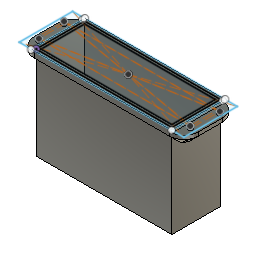
Aerostar Dash Bin Cubby v3 (Autodesk Fusion 360 design; units mm, degrees)
Autodesk Fusion 360 part; units mm, degrees
sketch "Sketch1" plane through (0, 0, 0) normal (0, 0, 1) x (1, 0, 0)
  line L0 (0, 0) -> (183, 0)
  line L1 (183, 0) -> (183, 65.4)
  line L2 (183, 65.4) -> (0, 65.4)
  line L3 (0, 65.4) -> (0, 0)
  line L4 (3.3, 62.1) -> (3.3, 3.3)
  line L5 (3.3, 3.3) -> (179.7, 3.3)
  line L6 (179.7, 3.3) -> (179.7, 62.1)
  line L7 (179.7, 62.1) -> (3.3, 62.1)
  line L8 (196.5, 51.2) -> (-13.5, 51.2) construction
  line L9 (-13.5, 51.2) -> (-13.5, 14.2) construction
  line L10 (-13.5, 14.2) -> (196.5, 14.2) construction
  line L11 (196.5, 14.2) -> (196.5, 51.2) construction
  line L12 (196.5, 51.2) -> (-13.5, 14.2) construction
  line L13 (-13.5, 51.2) -> (196.5, 14.2) construction
  line L14 (193.5, 51.2) -> (-10.5, 51.2) construction
  line L15 (-10.5, 51.2) -> (-10.5, 14.2) construction
  line L16 (-10.5, 14.2) -> (193.5, 14.2) construction
  line L17 (193.5, 14.2) -> (193.5, 51.2) construction
  line L18 (193.5, 51.2) -> (-10.5, 14.2) construction
  line L19 (-10.5, 51.2) -> (193.5, 14.2) construction
  circle A0 centre (-13.5, 51.2) radius 3.1
  circle A1 centre (196.5, 51.2) radius 3.1
  circle A2 centre (-10.5, 14.2) radius 3.1
  circle A3 centre (193.5, 14.2) radius 3.1
  line L20 (183, 65.4) -> (186, 65.4) construction
  line L21 (0, 65.4) -> (-3, 65.4) construction
  line L22 (186, 68.7) -> (186, -3.3)
  line L23 (-3, 68.7) -> (-3, -4)
  line L24 (202.5, 68.7) -> (-19.5, 68.7)
  line L25 (-19.5, 68.7) -> (-19.5, -3.3)
  line L26 (-19.5, -3.3) -> (202.5, -3.3)
  line L27 (202.5, -3.3) -> (202.5, 68.7)
  line L28 (202.5, 68.7) -> (-19.5, -3.3) construction
  line L29 (-19.5, 68.7) -> (202.5, -3.3) construction
  point P0 (91.5, 32.7)
  point P1 (91.5, 32.7)
  point P2 (91.5, 32.7)
  point P3 (91.5, 32.7)
  dimension "d1" = 65.4
  dimension "d2" = 183
  dimension "d3" = 3.3
  dimension "d4" = 37
  dimension "d5" = 204
  dimension "d6" = 6.2
  dimension "d7" = 6.2
  dimension "d8" = 6.2
  dimension "d9" = 6.2
  dimension "d20" = 3
  dimension "d21" = 3
  dimension "d26" = 222
  dimension "d27" = 72
  constraint horizontal L0
  constraint vertical L1
  constraint horizontal L2
  constraint vertical L3
  constraint coincident L0.start L3.end
  constraint perpendicular L8 L9
  constraint parallel L8 L10
  constraint parallel L9 L11
  constraint horizontal L8
  constraint coincident L12 P3
  constraint coincident L13 P3
  constraint perpendicular L14 L15
  constraint parallel L14 L16
  constraint parallel L15 L17
  constraint horizontal L14
  constraint coincident L18 P3
  constraint coincident L19 P3
  constraint coincident P3 P2
  constraint coincident L8.end L9.start
  constraint coincident L8.start L11.end
  constraint coincident L15.end L16.start
  constraint coincident L16.end L17.start
  constraint perpendicular L24 L25
  constraint parallel L24 L26
  constraint parallel L25 L27
  constraint horizontal L24
  constraint coincident L28 P3
  constraint coincident L29 P3
  measures "d1" distance of L0.start L2.end
  measures "d2" distance of L0.start L0.end
  measures "d4" distance of L8.end L9.end
  measures "d5" distance of L15.end L16.end
  measures "d6" diameter of A0
  measures "d7" diameter of A1
  measures "d8" diameter of A2
  measures "d9" diameter of A3
  measures "d20" distance of L1.end L20.end
  measures "d21" distance of L2.end L21.end
  measures "d26" distance of L25.end L26.end
  measures "d27" distance of L24.end L25.end
extrude "Extrude1" add sketch "Sketch1" against normal blind 125 contours L0 L1 L2 L3
extrude "Extrude2" add sketch "Sketch1" against normal blind 7.4 contours L22 L24 L26 L27 | L22 L23 L24 L26 | L23 L24 L25 L26
extrude "Extrude3" cut sketch "Sketch1" against normal blind 3.5 contours A0 | A2 | L22 L24 L26 L27 | L23 L24 L25 L26
sketch "Sketch2" plane through (0, 0, -125) normal (0, 0, -1) x (1, 0, 0)
  line L0 (179.7, -62.1) -> (3.3, -62.1)
  line L1 (3.3, -62.1) -> (3.3, -3.3)
  line L2 (3.3, -3.3) -> (179.7, -3.3)
  line L3 (179.7, -3.3) -> (179.7, -62.1)
  line L4 (0, 0) -> (0, -65.4)
  line L5 (0, -65.4) -> (183, -65.4)
  line L6 (183, -65.4) -> (183, 0)
  line L7 (183, 0) -> (0, 0)
  line L8 (3.3, -62.1) -> (3.3, -3.3)
  line L9 (3.3, -3.3) -> (179.7, -3.3)
  line L10 (179.7, -62.1) -> (3.3, -62.1)
  line L11 (179.7, -3.3) -> (179.7, -62.1)
extrude "Extrude4" add sketch "Sketch2" against normal blind 3.3 contours L0 L1 L2 L3 L8 L9 L10 L11
fillet "Fillet1" radius 20 4 edges at (202.5, 68.7, -5.45) (202.5, -3.3, -5.45) (-19.5, 68.7, -5.45) (-19.5, -3.3, -5.45)
extrude "Extrude5" add 1 faces at (189.1588, 43.8775, -7.4) along direction (0, 0, -1) blind 15
sketch "Sketch3" plane through (0, 0, -22.4) normal (0, 0, -1) x (1, 0, 0)
  arc A0 (0.5, 3.3) -> (-19.5, -16.7) centre (0.5, -16.7) ccw
  line L0 (-19.5, -16.7) -> (-19.5, -48.7)
  arc A1 (-19.5, -48.7) -> (0.5, -68.7) centre (0.5, -48.7) ccw
  line L1 (0.5, -68.7) -> (182.5, -68.7)
  arc A2 (182.5, -68.7) -> (202.5, -48.7) centre (182.5, -48.7) ccw
  line L2 (202.5, -48.7) -> (202.5, -16.7)
  arc A3 (202.5, -16.7) -> (182.5, 3.3) centre (182.5, -16.7) ccw
  line L3 (182.5, 3.3) -> (0.5, 3.3)
  circle A4 centre (196.5, -51.2) radius 3.1
  line L4 (0, -65.4) -> (0, 0)
  line L5 (0, 0) -> (183, 0)
  line L6 (183, 0) -> (183, -65.4)
  line L7 (183, -65.4) -> (0, -65.4)
  circle A5 centre (-13.5, -51.2) radius 3.1
  circle A6 centre (193.5, -14.2) radius 3.1
  circle A7 centre (-10.5, -14.2) radius 3.1
  circle A8 centre (196.5, -51.2) radius 6.5
  circle A9 centre (193.5, -14.2) radius 6.5
  circle A10 centre (-10.5, -14.2) radius 6.5
  circle A11 centre (-13.5, -51.2) radius 6.5
  dimension "d31" = 13
  dimension "d32" = 13
  dimension "d33" = 13
  dimension "d34" = 13
  constraint concentric A4 A8
  constraint concentric A6 A9
  constraint concentric A7 A10
  constraint concentric A5 A11
  measures "d31" diameter of A8
  measures "d32" diameter of A9
  measures "d33" diameter of A10
  measures "d34" diameter of A11
extrude "Extrude6" cut sketch "Sketch3" against normal blind 13 contours A1 A11 | A2 A8 | A9 | A10 picked at (-18.4412, -50.0123) picked at (201.4412, -50.0123)
chamfer "Chamfer1" distance 14 distance2 14 8 edges at (202.5, 32.7, -22.4) (196.6421, 2.5579, -22.4) (91.5, -3.3, -22.4) (-13.6421, 2.5579, -22.4) (-19.5, 32.7, -22.4) (-10.9359, 65.108, -22.4) (91.5, 68.7, -22.4) (193.9359, 65.108, -22.4) measured on face at (186.9487, 44.0037, -22.4) measured on face at (186.9487, 44.0037, -22.4) measured on face at (186.9487, 44.0037, -22.4) measured on face at (186.9487, 44.0037, -22.4) measured on face at (186.9487, 44.0037, -22.4) measured on face at (186.9487, 44.0037, -22.4) measured on face at (186.9487, 44.0037, -22.4) measured on face at (186.9487, 44.0037, -22.4)
equation "d3 = 7 mm - 3.7 mm"
